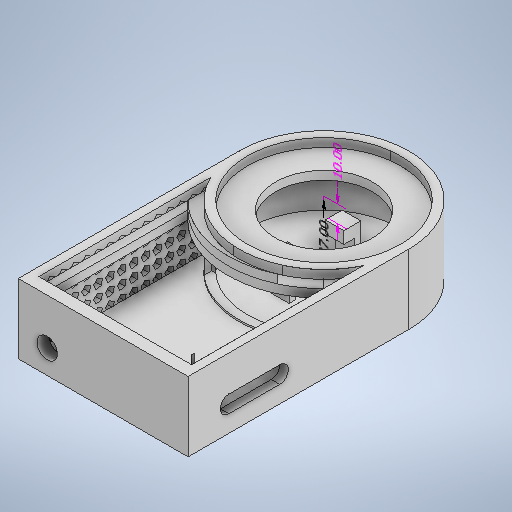
# Autodesk Inventor part: bazav2
Saved by Autodesk Inventor 2025.2 (Build 292293000, 293)
## iProperties
Created: 2025-08-28
Part Number: bazav2
Material: Ogólny
Document SubType Name: Modeling
Designer: IGOR
Density: 1 g/cm^3
Appearance: Domyślna
Author: IGOR
Autodesk Inventor part; units mm, degrees
ref_plane "YZ Plane" through (0, 0, 0) normal (1, 0, 0) x (0, 1, 0)
ref_plane "XZ Plane" through (0, 0, 0) normal (0, 1, 0) x (-1, 0, 0)
ref_plane "XY Plane" through (0, 0, 0) normal (0, 0, 1) x (1, 0, 0)
sketch "Szkic1" plane through (0, 0, 0) normal (0, 1, 0) x (-1, 0, 0)
  circle A0 centre (0.082273, -0.020568) radius 50
  circle A1 centre (0.082273, -0.020568) radius 45
  line L0 (-5.417727, 25.979432) -> (5.582273, 25.979432)
  line L1 (5.582273, 25.979432) -> (5.582273, 15.979432)
  line L2 (5.582273, 15.979432) -> (-5.417727, 15.979432)
  line L3 (-5.417727, 15.979432) -> (-5.417727, 25.979432)
  line L4 (-5.417727, 25.979432) -> (5.582273, 15.979432) construction
  line L5 (5.582273, 25.979432) -> (-5.417727, 15.979432) construction
  line L6 (-5.417727, -6.270568) -> (5.582273, -6.270568)
  line L7 (5.582273, -6.270568) -> (5.582273, -16.270568)
  line L8 (5.582273, -16.270568) -> (-5.417727, -16.270568)
  line L9 (-5.417727, -16.270568) -> (-5.417727, -6.270568)
  line L10 (-5.417727, -6.270568) -> (5.582273, -16.270568) construction
  line L11 (5.582273, -6.270568) -> (-5.417727, -16.270568) construction
  line L12 (50.082273, -0.020568) -> (50.082273, 129.979432)
  line L13 (50.082273, 129.979432) -> (-49.917727, 129.979432)
  line L14 (-49.917727, 129.979432) -> (-49.917727, -0.020568)
  line L15 (-17.866681, -46.687849) -> (50.082273, 129.979432) construction
  line L16 (18.031227, -46.687849) -> (-49.917727, 129.979432) construction
  line L17 (45.082273, -21.815063) -> (45.082273, 123)
  line L18 (45.082273, 123) -> (-44.917727, 123)
  line L19 (-44.917727, 123) -> (-44.917727, -21.815063)
  line L20 (-17.09427, -46.977638) -> (45.082273, 123) construction
  line L21 (17.258816, -46.977638) -> (-44.917727, 123) construction
  point P0 (0, 0)
  point P1 (0.082273, 20.979432)
  point P2 (0.082273, -11.270568)
  point P3 (0.082273, 15.979432)
  point P4 (45.082273, 21.773926)
  point P5 (-44.917727, 21.773926)
  dimension "d0" = 100
  dimension "d1" = 90
  dimension "d2" = 11
  dimension "d3" = 10
  dimension "d4" = 11
  dimension "d5" = 10
  dimension "d6" = 6.25
  dimension "d7" = 16
  constraints: 44 end point, 6 parallel, 5 midpoint, 4 point on line, 2 coincident, 2 horizontal, 2 perpendicular, 1 centre point, 10 other
  measures "d1" diameter of A1
  measures "d2" distance of L2.start L2.end
  measures "d3" distance of L5.start L2.start
  measures "d4" distance of L7.end L9.start
  measures "d5" distance of L6.end L7.end
  measures "d6" distance from line of point (0.082, -0.021) L6
  measures "d7" distance of point (0.082, 15.979) point (0.082, -0.021)
extrude "Wyciągnięcie proste1" add sketch "Szkic1" along normal blind 41 contours A0 L19 | L14 L13 L12 A0 L17 L18 L19 | L19 A1 L17 A0 | A0 L17 A1 L19 | L17 A0
extrude "Wyciągnięcie proste2" add sketch "Szkic1" along normal blind 4 contours L19 L18 L17 A0 | A1
extrude "Wyciągnięcie proste3" add sketch "Szkic1" along normal blind 25 contours L0 L1 L2 L3 | L6 L7 L8 L9
sketch "Szkic2" plane through (44.917727, 41, 123) normal (0, 0, -1) x (-1, 0, 0)
  line L0 (78, -36) -> (6, -36)
  line L1 (6, -36) -> (6, -10)
  line L2 (6, -10) -> (78, -10)
  line L3 (78, -10) -> (78, -36)
  point P0 (44.917727, -41)
  constraints: 8 end point, 2 parallel, 1 horizontal, 1 perpendicular
extrude "Wyciągnięcie proste4" cut sketch "Szkic2" along normal blind 90
sketch "Szkic3" plane through (0, 41, 0) normal (0, 1, 0) x (1, 0, 0)
  circle A0 centre (0, 0) radius 45.009943
  circle A1 centre (0, 0) radius 28.551038
  constraints: 2 centre point, 2 coincident
extrude "Wyciągnięcie proste5" add sketch "Szkic3" against normal blind 10
sketch "Szkic4" plane through (0, 41, 0) normal (0, 1, 0) x (1, 0, 0)
  circle A0 centre (0, 0) radius 45.03064
  circle A1 centre (0, 0) radius 28.551038
  constraints: 2 centre point, 2 coincident
extrude "Wyciągnięcie proste6" cut sketch "Szkic4" against normal blind 5
sketch "Szkic5" plane through (5.417727, 4, -16.270568) normal (1, 0, 0) x (0, 0, -1)
  line L0 (0, 0) -> (-10, 0) projected
  line L1 (-10, 0) -> (-4, 0)
  line L2 (-4, 0) -> (-4, 14)
  line L3 (-4, 14) -> (-10, 14)
  line L4 (-10, 14) -> (-10, 0)
  line L5 (-32.25, 0) -> (-42.25, 0) projected
  line L6 (-32.25, 0) -> (-38.25, 0)
  line L7 (-38.25, 0) -> (-38.25, 14)
  line L8 (-38.25, 14) -> (-32.25, 14)
  line L9 (-32.25, 14) -> (-32.25, 0)
  point P0 (-16.270568, -4)
  point P1 (-4, 0)
  point P2 (-38.25, 0)
  dimension "d23" = 6
  dimension "d24" = 14
  constraints: 16 end point, 4 parallel, 2 horizontal, 2 perpendicular
  measures "d23" distance of L7.end L8.end
  measures "d24" distance of L6.end L7.end
extrude "Wyciągnięcie proste7" cut sketch "Szkic5" against normal blind 11
sketch "Szkic6" plane through (0, 41, 0) normal (0, 1, 0) x (1, 0, 0)
  line L0 (44.917727, -21.773926) -> (44.917727, -123)
  line L1 (-45.082273, -123) -> (44.917727, -123)
  line L2 (44.917727, -123) -> (44.917727, -21.773926)
  line L3 (-45.025483, -21.773926) -> (-45.082273, -21.773926)
  line L4 (-45.082273, -21.773926) -> (-45.082273, -123)
  arc A0 (-45.025483, -21.773926) -> (44.917727, -21.995359) centre (0, 0) ccw
  arc A1 (-40.082273, -40.132904) -> (39.917727, -40.296572) centre (0, 0) ccw
  line L5 (-40.082273, -118) -> (39.917727, -118)
  line L6 (39.917727, -118) -> (39.917727, -40.296572)
  line L7 (-40.082273, -40.132904) -> (-40.082273, -118)
  point P0 (39.917727, -79.148286)
  point P1 (44.917727, -21.995359)
  dimension "d27" = 5
  dimension "d28" = 5
  dimension "d29" = 5
  dimension "d30" = 6.70673
  constraints: 14 end point, 4 point on circle, 3 parallel, 2 centre point, 2 coincident, 2 horizontal, 2 perpendicular, 1 midpoint, 1 point on line
  measures "d27" distance from line of point (39.918, -79.148) L0
  measures "d28" distance between parallel lines of L4 L7
  measures "d29" distance between parallel lines of L1 L5
  measures "d30" radial gap between concentric circles of A1 A0
extrude "Wyciągnięcie proste8" add sketch "Szkic6" against normal blind 10
sketch "Szkic7" plane through (0, 41, 0) normal (0, 1, 0) x (1, 0, 0)
  line L0 (44.972521, -21.748488) -> (44.972521, -122.974561)
  line L1 (-45.027479, -122.974561) -> (44.972521, -122.974561)
  line L2 (44.972521, -122.974561) -> (44.972521, -21.748488)
  line L3 (-44.970689, -21.748488) -> (-45.027479, -21.748488)
  line L4 (-45.027479, -21.748488) -> (-45.027479, -122.974561)
  arc A0 (-44.970689, -21.748488) -> (44.972521, -21.96992) centre (0.054794, 0.025439) ccw
  arc A1 (-40.027479, -40.107466) -> (39.972521, -40.271133) centre (0.054794, 0.025439) ccw
  line L5 (-40.027479, -117.974561) -> (39.972521, -117.974561)
  line L6 (39.972521, -117.974561) -> (39.972521, -40.271133)
  line L7 (-40.027479, -40.107466) -> (-40.027479, -117.974561)
  point P0 (0, 0)
  point P1 (39.972521, -79.122847)
  point P2 (44.972521, -21.96992)
  dimension "d33" = 5
  dimension "d34" = 5
  dimension "d35" = 5
  dimension "d36" = 6.70673
  constraints: 16 end point, 4 point on circle, 3 parallel, 2 centre point, 2 horizontal, 2 perpendicular, 1 coincident, 1 midpoint, 1 point on line
  measures "d33" distance from line of point (39.973, -79.123) L0
  measures "d34" distance between parallel lines of L4 L7
  measures "d35" distance between parallel lines of L1 L5
  measures "d36" radial gap between concentric circles of A1 A0
extrude "Wyciągnięcie proste9" cut sketch "Szkic7" against normal blind 5
sketch "Szkic8" plane through (39.917727, 31, 40.296572) normal (-1, 0, 0) x (0, 0, 1)
  line L0 (0.028766, 10) -> (77.677989, 10)
  line L1 (0, 5) -> (0, 0)
  line L2 (76, 10) -> (0, 10)
  line L3 (0, 10) -> (0, 5)
  line L4 (0, 5) -> (76, 5)
  line L5 (76, 5) -> (76, 10)
  point P0 (-40.296572, -31)
  constraints: 8 end point, 2 parallel, 1 horizontal, 1 perpendicular, 1 point on line
extrude "Wyciągnięcie proste10" cut sketch "Szkic8" against normal blind 1
sketch "Szkic9" plane through (-50.082273, 0, 129.979432) normal (0, 0, 1) x (1, 0, 0)
  line L0 (17, 5) -> (17, 31) projected
  circle A0 centre (17, 14) radius 6
  point P0 (50.082273, 0)
  dimension "d41" = 12
  constraints: 1 centre point, 1 point on line
  measures "d41" diameter of A0
extrude "Wyciągnięcie proste11" cut sketch "Szkic9" against normal blind 10
sketch "Szkic11" plane through (49.917727, 0, 129.979432) normal (1, 0, 0) x (0, 0, -1)
  line L0 (24, 15) -> (54, 15) construction
  line L1 (24, 10) -> (54, 10)
  line L2 (54, 20) -> (24, 20)
  arc A0 (24, 20) -> (24, 10) centre (24, 15) ccw
  arc A1 (54, 10) -> (54, 20) centre (54, 15) ccw
  point P0 (129.979432, 0)
  point P1 (39, 15)
  constraints: 8 end point, 4 point on circle, 4 tangent, 2 centre point, 1 horizontal, 1 midpoint, 1 parallel
extrude "Wyciągnięcie proste13" cut sketch "Szkic11" against normal blind 10
sketch "Szkic12" plane through (-50.082273, 0, -0.020568) normal (-1, 0, 0) x (0, 0, 1)
  line L0 (12.273457, 32.546915) -> (9.060497, 33.030825)
  line L1 (9.060497, 33.030825) -> (8.527864, 36.236068)
  line L2 (8.527864, 36.236068) -> (11.411638, 37.733107)
  line L3 (11.411638, 37.733107) -> (13.726543, 35.453085)
  line L4 (13.726543, 35.453085) -> (12.273457, 32.546915)
  line L5 (0, 0) -> (0, 41)
  line L6 (130, 0) -> (130, 41)
  line L7 (0, 41) -> (130, 41)
  line L8 (130, 41) -> (130, 0)
  line L9 (130, 0) -> (0, 0)
  line L10 (0, 0) -> (0, 41)
  line L11 (18.411638, 37.733107) -> (20.726543, 35.453085)
  line L12 (20.726543, 35.453085) -> (19.273457, 32.546915)
  line L13 (19.273457, 32.546915) -> (16.060497, 33.030825)
  line L14 (16.060497, 33.030825) -> (15.527864, 36.236068)
  line L15 (15.527864, 36.236068) -> (18.411638, 37.733107)
  line L16 (25.411638, 37.733107) -> (27.726543, 35.453085)
  line L17 (27.726543, 35.453085) -> (26.273457, 32.546915)
  line L18 (26.273457, 32.546915) -> (23.060497, 33.030825)
  line L19 (23.060497, 33.030825) -> (22.527864, 36.236068)
  line L20 (22.527864, 36.236068) -> (25.411638, 37.733107)
  line L21 (32.411638, 37.733107) -> (34.726543, 35.453085)
  line L22 (34.726543, 35.453085) -> (33.273457, 32.546915)
  line L23 (33.273457, 32.546915) -> (30.060497, 33.030825)
  line L24 (30.060497, 33.030825) -> (29.527864, 36.236068)
  line L25 (29.527864, 36.236068) -> (32.411638, 37.733107)
  line L26 (39.411638, 37.733107) -> (41.726543, 35.453085)
  line L27 (41.726543, 35.453085) -> (40.273457, 32.546915)
  line L28 (40.273457, 32.546915) -> (37.060497, 33.030825)
  line L29 (37.060497, 33.030825) -> (36.527864, 36.236068)
  line L30 (36.527864, 36.236068) -> (39.411638, 37.733107)
  line L31 (46.411638, 37.733107) -> (48.726543, 35.453085)
  line L32 (48.726543, 35.453085) -> (47.273457, 32.546915)
  line L33 (47.273457, 32.546915) -> (44.060497, 33.030825)
  line L34 (44.060497, 33.030825) -> (43.527864, 36.236068)
  line L35 (43.527864, 36.236068) -> (46.411638, 37.733107)
  line L36 (53.411638, 37.733107) -> (55.726543, 35.453085)
  line L37 (55.726543, 35.453085) -> (54.273457, 32.546915)
  line L38 (54.273457, 32.546915) -> (51.060497, 33.030825)
  line L39 (51.060497, 33.030825) -> (50.527864, 36.236068)
  line L40 (50.527864, 36.236068) -> (53.411638, 37.733107)
  line L41 (60.411638, 37.733107) -> (62.726543, 35.453085)
  line L42 (62.726543, 35.453085) -> (61.273457, 32.546915)
  line L43 (61.273457, 32.546915) -> (58.060497, 33.030825)
  line L44 (58.060497, 33.030825) -> (57.527864, 36.236068)
  line L45 (57.527864, 36.236068) -> (60.411638, 37.733107)
  line L46 (67.411638, 37.733107) -> (69.726543, 35.453085)
  line L47 (69.726543, 35.453085) -> (68.273457, 32.546915)
  line L48 (68.273457, 32.546915) -> (65.060497, 33.030825)
  line L49 (65.060497, 33.030825) -> (64.527864, 36.236068)
  line L50 (64.527864, 36.236068) -> (67.411638, 37.733107)
  line L51 (74.411638, 37.733107) -> (76.726543, 35.453085)
  line L52 (76.726543, 35.453085) -> (75.273457, 32.546915)
  line L53 (75.273457, 32.546915) -> (72.060497, 33.030825)
  line L54 (72.060497, 33.030825) -> (71.527864, 36.236068)
  line L55 (71.527864, 36.236068) -> (74.411638, 37.733107)
  line L56 (81.411638, 37.733107) -> (83.726543, 35.453085)
  line L57 (83.726543, 35.453085) -> (82.273457, 32.546915)
  line L58 (82.273457, 32.546915) -> (79.060497, 33.030825)
  line L59 (79.060497, 33.030825) -> (78.527864, 36.236068)
  line L60 (78.527864, 36.236068) -> (81.411638, 37.733107)
  line L61 (88.411638, 37.733107) -> (90.726543, 35.453085)
  line L62 (90.726543, 35.453085) -> (89.273457, 32.546915)
  line L63 (89.273457, 32.546915) -> (86.060497, 33.030825)
  line L64 (86.060497, 33.030825) -> (85.527864, 36.236068)
  line L65 (85.527864, 36.236068) -> (88.411638, 37.733107)
  line L66 (95.411638, 37.733107) -> (97.726543, 35.453085)
  line L67 (97.726543, 35.453085) -> (96.273457, 32.546915)
  line L68 (96.273457, 32.546915) -> (93.060497, 33.030825)
  line L69 (93.060497, 33.030825) -> (92.527864, 36.236068)
  line L70 (92.527864, 36.236068) -> (95.411638, 37.733107)
  line L71 (102.411638, 37.733107) -> (104.726543, 35.453085)
  line L72 (104.726543, 35.453085) -> (103.273457, 32.546915)
  line L73 (103.273457, 32.546915) -> (100.060497, 33.030825)
  line L74 (100.060497, 33.030825) -> (99.527864, 36.236068)
  line L75 (99.527864, 36.236068) -> (102.411638, 37.733107)
  line L76 (109.411638, 37.733107) -> (111.726543, 35.453085)
  line L77 (111.726543, 35.453085) -> (110.273457, 32.546915)
  line L78 (110.273457, 32.546915) -> (107.060497, 33.030825)
  line L79 (107.060497, 33.030825) -> (106.527864, 36.236068)
  line L80 (106.527864, 36.236068) -> (109.411638, 37.733107)
  line L81 (116.411638, 37.733107) -> (118.726543, 35.453085)
  line L82 (118.726543, 35.453085) -> (117.273457, 32.546915)
  line L83 (117.273457, 32.546915) -> (114.060497, 33.030825)
  line L84 (114.060497, 33.030825) -> (113.527864, 36.236068)
  line L85 (113.527864, 36.236068) -> (116.411638, 37.733107)
  line L86 (123.411638, 37.733107) -> (125.726543, 35.453085)
  line L87 (125.726543, 35.453085) -> (124.273457, 32.546915)
  line L88 (124.273457, 32.546915) -> (121.060497, 33.030825)
  line L89 (121.060497, 33.030825) -> (120.527864, 36.236068)
  line L90 (120.527864, 36.236068) -> (123.411638, 37.733107)
  line L91 (11.411638, 30.233107) -> (13.726543, 27.953085)
  line L92 (13.726543, 27.953085) -> (12.273457, 25.046915)
  line L93 (12.273457, 25.046915) -> (9.060497, 25.530825)
  line L94 (9.060497, 25.530825) -> (8.527864, 28.736068)
  line L95 (8.527864, 28.736068) -> (11.411638, 30.233107)
  line L96 (18.411638, 30.233107) -> (20.726543, 27.953085)
  line L97 (20.726543, 27.953085) -> (19.273457, 25.046915)
  line L98 (19.273457, 25.046915) -> (16.060497, 25.530825)
  line L99 (16.060497, 25.530825) -> (15.527864, 28.736068)
  line L100 (15.527864, 28.736068) -> (18.411638, 30.233107)
  line L101 (25.411638, 30.233107) -> (27.726543, 27.953085)
  line L102 (27.726543, 27.953085) -> (26.273457, 25.046915)
  line L103 (26.273457, 25.046915) -> (23.060497, 25.530825)
  line L104 (23.060497, 25.530825) -> (22.527864, 28.736068)
  line L105 (22.527864, 28.736068) -> (25.411638, 30.233107)
  line L106 (32.411638, 30.233107) -> (34.726543, 27.953085)
  line L107 (34.726543, 27.953085) -> (33.273457, 25.046915)
  line L108 (33.273457, 25.046915) -> (30.060497, 25.530825)
  line L109 (30.060497, 25.530825) -> (29.527864, 28.736068)
  line L110 (29.527864, 28.736068) -> (32.411638, 30.233107)
  line L111 (39.411638, 30.233107) -> (41.726543, 27.953085)
  line L112 (41.726543, 27.953085) -> (40.273457, 25.046915)
  line L113 (40.273457, 25.046915) -> (37.060497, 25.530825)
  line L114 (37.060497, 25.530825) -> (36.527864, 28.736068)
  line L115 (36.527864, 28.736068) -> (39.411638, 30.233107)
  line L116 (46.411638, 30.233107) -> (48.726543, 27.953085)
  line L117 (48.726543, 27.953085) -> (47.273457, 25.046915)
  line L118 (47.273457, 25.046915) -> (44.060497, 25.530825)
  line L119 (44.060497, 25.530825) -> (43.527864, 28.736068)
  line L120 (43.527864, 28.736068) -> (46.411638, 30.233107)
  line L121 (53.411638, 30.233107) -> (55.726543, 27.953085)
  line L122 (55.726543, 27.953085) -> (54.273457, 25.046915)
  line L123 (54.273457, 25.046915) -> (51.060497, 25.530825)
  line L124 (51.060497, 25.530825) -> (50.527864, 28.736068)
  line L125 (50.527864, 28.736068) -> (53.411638, 30.233107)
  line L126 (60.411638, 30.233107) -> (62.726543, 27.953085)
  line L127 (62.726543, 27.953085) -> (61.273457, 25.046915)
  line L128 (61.273457, 25.046915) -> (58.060497, 25.530825)
  line L129 (58.060497, 25.530825) -> (57.527864, 28.736068)
  line L130 (57.527864, 28.736068) -> (60.411638, 30.233107)
  line L131 (67.411638, 30.233107) -> (69.726543, 27.953085)
  line L132 (69.726543, 27.953085) -> (68.273457, 25.046915)
  line L133 (68.273457, 25.046915) -> (65.060497, 25.530825)
  line L134 (65.060497, 25.530825) -> (64.527864, 28.736068)
  line L135 (64.527864, 28.736068) -> (67.411638, 30.233107)
  line L136 (74.411638, 30.233107) -> (76.726543, 27.953085)
  line L137 (76.726543, 27.953085) -> (75.273457, 25.046915)
  line L138 (75.273457, 25.046915) -> (72.060497, 25.530825)
  line L139 (72.060497, 25.530825) -> (71.527864, 28.736068)
  line L140 (71.527864, 28.736068) -> (74.411638, 30.233107)
  line L141 (81.411638, 30.233107) -> (83.726543, 27.953085)
  line L142 (83.726543, 27.953085) -> (82.273457, 25.046915)
  line L143 (82.273457, 25.046915) -> (79.060497, 25.530825)
  line L144 (79.060497, 25.530825) -> (78.527864, 28.736068)
  line L145 (78.527864, 28.736068) -> (81.411638, 30.233107)
  line L146 (88.411638, 30.233107) -> (90.726543, 27.953085)
  line L147 (90.726543, 27.953085) -> (89.273457, 25.046915)
  line L148 (89.273457, 25.046915) -> (86.060497, 25.530825)
  line L149 (86.060497, 25.530825) -> (85.527864, 28.736068)
  line L150 (85.527864, 28.736068) -> (88.411638, 30.233107)
  line L151 (95.411638, 30.233107) -> (97.726543, 27.953085)
  line L152 (97.726543, 27.953085) -> (96.273457, 25.046915)
  line L153 (96.273457, 25.046915) -> (93.060497, 25.530825)
  line L154 (93.060497, 25.530825) -> (92.527864, 28.736068)
  line L155 (92.527864, 28.736068) -> (95.411638, 30.233107)
  line L156 (102.411638, 30.233107) -> (104.726543, 27.953085)
  line L157 (104.726543, 27.953085) -> (103.273457, 25.046915)
  line L158 (103.273457, 25.046915) -> (100.060497, 25.530825)
  line L159 (100.060497, 25.530825) -> (99.527864, 28.736068)
  line L160 (99.527864, 28.736068) -> (102.411638, 30.233107)
  line L161 (109.411638, 30.233107) -> (111.726543, 27.953085)
  line L162 (111.726543, 27.953085) -> (110.273457, 25.046915)
  line L163 (110.273457, 25.046915) -> (107.060497, 25.530825)
  line L164 (107.060497, 25.530825) -> (106.527864, 28.736068)
  line L165 (106.527864, 28.736068) -> (109.411638, 30.233107)
  line L166 (116.411638, 30.233107) -> (118.726543, 27.953085)
  line L167 (118.726543, 27.953085) -> (117.273457, 25.046915)
  line L168 (117.273457, 25.046915) -> (114.060497, 25.530825)
  line L169 (114.060497, 25.530825) -> (113.527864, 28.736068)
  line L170 (113.527864, 28.736068) -> (116.411638, 30.233107)
  line L171 (123.411638, 30.233107) -> (125.726543, 27.953085)
  line L172 (125.726543, 27.953085) -> (124.273457, 25.046915)
  line L173 (124.273457, 25.046915) -> (121.060497, 25.530825)
  line L174 (121.060497, 25.530825) -> (120.527864, 28.736068)
  line L175 (120.527864, 28.736068) -> (123.411638, 30.233107)
  line L176 (11.411638, 22.733107) -> (13.726543, 20.453085)
  line L177 (13.726543, 20.453085) -> (12.273457, 17.546915)
  line L178 (12.273457, 17.546915) -> (9.060497, 18.030825)
  line L179 (9.060497, 18.030825) -> (8.527864, 21.236068)
  line L180 (8.527864, 21.236068) -> (11.411638, 22.733107)
  line L181 (18.411638, 22.733107) -> (20.726543, 20.453085)
  line L182 (20.726543, 20.453085) -> (19.273457, 17.546915)
  line L183 (19.273457, 17.546915) -> (16.060497, 18.030825)
  line L184 (16.060497, 18.030825) -> (15.527864, 21.236068)
  line L185 (15.527864, 21.236068) -> (18.411638, 22.733107)
  line L186 (25.411638, 22.733107) -> (27.726543, 20.453085)
  line L187 (27.726543, 20.453085) -> (26.273457, 17.546915)
  line L188 (26.273457, 17.546915) -> (23.060497, 18.030825)
  line L189 (23.060497, 18.030825) -> (22.527864, 21.236068)
  line L190 (22.527864, 21.236068) -> (25.411638, 22.733107)
  line L191 (32.411638, 22.733107) -> (34.726543, 20.453085)
  line L192 (34.726543, 20.453085) -> (33.273457, 17.546915)
  line L193 (33.273457, 17.546915) -> (30.060497, 18.030825)
  line L194 (30.060497, 18.030825) -> (29.527864, 21.236068)
  line L195 (29.527864, 21.236068) -> (32.411638, 22.733107)
  line L196 (39.411638, 22.733107) -> (41.726543, 20.453085)
  line L197 (41.726543, 20.453085) -> (40.273457, 17.546915)
  line L198 (40.273457, 17.546915) -> (37.060497, 18.030825)
  line L199 (37.060497, 18.030825) -> (36.527864, 21.236068)
  line L200 (36.527864, 21.236068) -> (39.411638, 22.733107)
  line L201 (46.411638, 22.733107) -> (48.726543, 20.453085)
  line L202 (48.726543, 20.453085) -> (47.273457, 17.546915)
  line L203 (47.273457, 17.546915) -> (44.060497, 18.030825)
  line L204 (44.060497, 18.030825) -> (43.527864, 21.236068)
  line L205 (43.527864, 21.236068) -> (46.411638, 22.733107)
  line L206 (53.411638, 22.733107) -> (55.726543, 20.453085)
  line L207 (55.726543, 20.453085) -> (54.273457, 17.546915)
  line L208 (54.273457, 17.546915) -> (51.060497, 18.030825)
  line L209 (51.060497, 18.030825) -> (50.527864, 21.236068)
  line L210 (50.527864, 21.236068) -> (53.411638, 22.733107)
  line L211 (60.411638, 22.733107) -> (62.726543, 20.453085)
  line L212 (62.726543, 20.453085) -> (61.273457, 17.546915)
  line L213 (61.273457, 17.546915) -> (58.060497, 18.030825)
  line L214 (58.060497, 18.030825) -> (57.527864, 21.236068)
  line L215 (57.527864, 21.236068) -> (60.411638, 22.733107)
  line L216 (67.411638, 22.733107) -> (69.726543, 20.453085)
  line L217 (69.726543, 20.453085) -> (68.273457, 17.546915)
  line L218 (68.273457, 17.546915) -> (65.060497, 18.030825)
  line L219 (65.060497, 18.030825) -> (64.527864, 21.236068)
  line L220 (64.527864, 21.236068) -> (67.411638, 22.733107)
  line L221 (74.411638, 22.733107) -> (76.726543, 20.453085)
  line L222 (76.726543, 20.453085) -> (75.273457, 17.546915)
  line L223 (75.273457, 17.546915) -> (72.060497, 18.030825)
  line L224 (72.060497, 18.030825) -> (71.527864, 21.236068)
  line L225 (71.527864, 21.236068) -> (74.411638, 22.733107)
  line L226 (81.411638, 22.733107) -> (83.726543, 20.453085)
  line L227 (83.726543, 20.453085) -> (82.273457, 17.546915)
  line L228 (82.273457, 17.546915) -> (79.060497, 18.030825)
  line L229 (79.060497, 18.030825) -> (78.527864, 21.236068)
  line L230 (78.527864, 21.236068) -> (81.411638, 22.733107)
  line L231 (88.411638, 22.733107) -> (90.726543, 20.453085)
  line L232 (90.726543, 20.453085) -> (89.273457, 17.546915)
  line L233 (89.273457, 17.546915) -> (86.060497, 18.030825)
  line L234 (86.060497, 18.030825) -> (85.527864, 21.236068)
  line L235 (85.527864, 21.236068) -> (88.411638, 22.733107)
  line L236 (95.411638, 22.733107) -> (97.726543, 20.453085)
  line L237 (97.726543, 20.453085) -> (96.273457, 17.546915)
  line L238 (96.273457, 17.546915) -> (93.060497, 18.030825)
  line L239 (93.060497, 18.030825) -> (92.527864, 21.236068)
  line L240 (92.527864, 21.236068) -> (95.411638, 22.733107)
  line L241 (102.411638, 22.733107) -> (104.726543, 20.453085)
  line L242 (104.726543, 20.453085) -> (103.273457, 17.546915)
  line L243 (103.273457, 17.546915) -> (100.060497, 18.030825)
  line L244 (100.060497, 18.030825) -> (99.527864, 21.236068)
  line L245 (99.527864, 21.236068) -> (102.411638, 22.733107)
  line L246 (109.411638, 22.733107) -> (111.726543, 20.453085)
  line L247 (111.726543, 20.453085) -> (110.273457, 17.546915)
  line L248 (110.273457, 17.546915) -> (107.060497, 18.030825)
  line L249 (107.060497, 18.030825) -> (106.527864, 21.236068)
  line L250 (106.527864, 21.236068) -> (109.411638, 22.733107)
  line L251 (116.411638, 22.733107) -> (118.726543, 20.453085)
  line L252 (118.726543, 20.453085) -> (117.273457, 17.546915)
  line L253 (117.273457, 17.546915) -> (114.060497, 18.030825)
  line L254 (114.060497, 18.030825) -> (113.527864, 21.236068)
  line L255 (113.527864, 21.236068) -> (116.411638, 22.733107)
  line L256 (123.411638, 22.733107) -> (125.726543, 20.453085)
  line L257 (125.726543, 20.453085) -> (124.273457, 17.546915)
  line L258 (124.273457, 17.546915) -> (121.060497, 18.030825)
  line L259 (121.060497, 18.030825) -> (120.527864, 21.236068)
  line L260 (120.527864, 21.236068) -> (123.411638, 22.733107)
  line L261 (11.411638, 15.233107) -> (13.726543, 12.953085)
  line L262 (13.726543, 12.953085) -> (12.273457, 10.046915)
  line L263 (12.273457, 10.046915) -> (9.060497, 10.530825)
  line L264 (9.060497, 10.530825) -> (8.527864, 13.736068)
  line L265 (8.527864, 13.736068) -> (11.411638, 15.233107)
  line L266 (18.411638, 15.233107) -> (20.726543, 12.953085)
  line L267 (20.726543, 12.953085) -> (19.273457, 10.046915)
  line L268 (19.273457, 10.046915) -> (16.060497, 10.530825)
  line L269 (16.060497, 10.530825) -> (15.527864, 13.736068)
  line L270 (15.527864, 13.736068) -> (18.411638, 15.233107)
  line L271 (25.411638, 15.233107) -> (27.726543, 12.953085)
  line L272 (27.726543, 12.953085) -> (26.273457, 10.046915)
  line L273 (26.273457, 10.046915) -> (23.060497, 10.530825)
  line L274 (23.060497, 10.530825) -> (22.527864, 13.736068)
  line L275 (22.527864, 13.736068) -> (25.411638, 15.233107)
  line L276 (32.411638, 15.233107) -> (34.726543, 12.953085)
  line L277 (34.726543, 12.953085) -> (33.273457, 10.046915)
  line L278 (33.273457, 10.046915) -> (30.060497, 10.530825)
  line L279 (30.060497, 10.530825) -> (29.527864, 13.736068)
  line L280 (29.527864, 13.736068) -> (32.411638, 15.233107)
  line L281 (39.411638, 15.233107) -> (41.726543, 12.953085)
  line L282 (41.726543, 12.953085) -> (40.273457, 10.046915)
  line L283 (40.273457, 10.046915) -> (37.060497, 10.530825)
  line L284 (37.060497, 10.530825) -> (36.527864, 13.736068)
  line L285 (36.527864, 13.736068) -> (39.411638, 15.233107)
  line L286 (46.411638, 15.233107) -> (48.726543, 12.953085)
  line L287 (48.726543, 12.953085) -> (47.273457, 10.046915)
  line L288 (47.273457, 10.046915) -> (44.060497, 10.530825)
  line L289 (44.060497, 10.530825) -> (43.527864, 13.736068)
  line L290 (43.527864, 13.736068) -> (46.411638, 15.233107)
  line L291 (53.411638, 15.233107) -> (55.726543, 12.953085)
  line L292 (55.726543, 12.953085) -> (54.273457, 10.046915)
  line L293 (54.273457, 10.046915) -> (51.060497, 10.530825)
  line L294 (51.060497, 10.530825) -> (50.527864, 13.736068)
  line L295 (50.527864, 13.736068) -> (53.411638, 15.233107)
  line L296 (60.411638, 15.233107) -> (62.726543, 12.953085)
  line L297 (62.726543, 12.953085) -> (61.273457, 10.046915)
  line L298 (61.273457, 10.046915) -> (58.060497, 10.530825)
  line L299 (58.060497, 10.530825) -> (57.527864, 13.736068)
  line L300 (57.527864, 13.736068) -> (60.411638, 15.233107)
  line L301 (67.411638, 15.233107) -> (69.726543, 12.953085)
  line L302 (69.726543, 12.953085) -> (68.273457, 10.046915)
  line L303 (68.273457, 10.046915) -> (65.060497, 10.530825)
  line L304 (65.060497, 10.530825) -> (64.527864, 13.736068)
  line L305 (64.527864, 13.736068) -> (67.411638, 15.233107)
  line L306 (74.411638, 15.233107) -> (76.726543, 12.953085)
  line L307 (76.726543, 12.953085) -> (75.273457, 10.046915)
  line L308 (75.273457, 10.046915) -> (72.060497, 10.530825)
  line L309 (72.060497, 10.530825) -> (71.527864, 13.736068)
  line L310 (71.527864, 13.736068) -> (74.411638, 15.233107)
  line L311 (81.411638, 15.233107) -> (83.726543, 12.953085)
  line L312 (83.726543, 12.953085) -> (82.273457, 10.046915)
  line L313 (82.273457, 10.046915) -> (79.060497, 10.530825)
  line L314 (79.060497, 10.530825) -> (78.527864, 13.736068)
  line L315 (78.527864, 13.736068) -> (81.411638, 15.233107)
  line L316 (88.411638, 15.233107) -> (90.726543, 12.953085)
  line L317 (90.726543, 12.953085) -> (89.273457, 10.046915)
  line L318 (89.273457, 10.046915) -> (86.060497, 10.530825)
  line L319 (86.060497, 10.530825) -> (85.527864, 13.736068)
  line L320 (85.527864, 13.736068) -> (88.411638, 15.233107)
  line L321 (95.411638, 15.233107) -> (97.726543, 12.953085)
  line L322 (97.726543, 12.953085) -> (96.273457, 10.046915)
  line L323 (96.273457, 10.046915) -> (93.060497, 10.530825)
  line L324 (93.060497, 10.530825) -> (92.527864, 13.736068)
  line L325 (92.527864, 13.736068) -> (95.411638, 15.233107)
  line L326 (102.411638, 15.233107) -> (104.726543, 12.953085)
  line L327 (104.726543, 12.953085) -> (103.273457, 10.046915)
  line L328 (103.273457, 10.046915) -> (100.060497, 10.530825)
  line L329 (100.060497, 10.530825) -> (99.527864, 13.736068)
  line L330 (99.527864, 13.736068) -> (102.411638, 15.233107)
  line L331 (109.411638, 15.233107) -> (111.726543, 12.953085)
  line L332 (111.726543, 12.953085) -> (110.273457, 10.046915)
  line L333 (110.273457, 10.046915) -> (107.060497, 10.530825)
  line L334 (107.060497, 10.530825) -> (106.527864, 13.736068)
  line L335 (106.527864, 13.736068) -> (109.411638, 15.233107)
  line L336 (116.411638, 15.233107) -> (118.726543, 12.953085)
  line L337 (118.726543, 12.953085) -> (117.273457, 10.046915)
  line L338 (117.273457, 10.046915) -> (114.060497, 10.530825)
  line L339 (114.060497, 10.530825) -> (113.527864, 13.736068)
  line L340 (113.527864, 13.736068) -> (116.411638, 15.233107)
  line L341 (123.411638, 15.233107) -> (125.726543, 12.953085)
  line L342 (125.726543, 12.953085) -> (124.273457, 10.046915)
  line L343 (124.273457, 10.046915) -> (121.060497, 10.530825)
  line L344 (121.060497, 10.530825) -> (120.527864, 13.736068)
  line L345 (120.527864, 13.736068) -> (123.411638, 15.233107)
  line L346 (11.411638, 7.733107) -> (13.726543, 5.453085)
  line L347 (13.726543, 5.453085) -> (12.273457, 2.546915)
  line L348 (12.273457, 2.546915) -> (9.060497, 3.030825)
  line L349 (9.060497, 3.030825) -> (8.527864, 6.236068)
  line L350 (8.527864, 6.236068) -> (11.411638, 7.733107)
  line L351 (18.411638, 7.733107) -> (20.726543, 5.453085)
  line L352 (20.726543, 5.453085) -> (19.273457, 2.546915)
  line L353 (19.273457, 2.546915) -> (16.060497, 3.030825)
  line L354 (16.060497, 3.030825) -> (15.527864, 6.236068)
  line L355 (15.527864, 6.236068) -> (18.411638, 7.733107)
  line L356 (25.411638, 7.733107) -> (27.726543, 5.453085)
  line L357 (27.726543, 5.453085) -> (26.273457, 2.546915)
  line L358 (26.273457, 2.546915) -> (23.060497, 3.030825)
  line L359 (23.060497, 3.030825) -> (22.527864, 6.236068)
  line L360 (22.527864, 6.236068) -> (25.411638, 7.733107)
  line L361 (32.411638, 7.733107) -> (34.726543, 5.453085)
  line L362 (34.726543, 5.453085) -> (33.273457, 2.546915)
  line L363 (33.273457, 2.546915) -> (30.060497, 3.030825)
  line L364 (30.060497, 3.030825) -> (29.527864, 6.236068)
  line L365 (29.527864, 6.236068) -> (32.411638, 7.733107)
  line L366 (39.411638, 7.733107) -> (41.726543, 5.453085)
  line L367 (41.726543, 5.453085) -> (40.273457, 2.546915)
  line L368 (40.273457, 2.546915) -> (37.060497, 3.030825)
  line L369 (37.060497, 3.030825) -> (36.527864, 6.236068)
  line L370 (36.527864, 6.236068) -> (39.411638, 7.733107)
  line L371 (46.411638, 7.733107) -> (48.726543, 5.453085)
  line L372 (48.726543, 5.453085) -> (47.273457, 2.546915)
  line L373 (47.273457, 2.546915) -> (44.060497, 3.030825)
  line L374 (44.060497, 3.030825) -> (43.527864, 6.236068)
  line L375 (43.527864, 6.236068) -> (46.411638, 7.733107)
  line L376 (53.411638, 7.733107) -> (55.726543, 5.453085)
  line L377 (55.726543, 5.453085) -> (54.273457, 2.546915)
  line L378 (54.273457, 2.546915) -> (51.060497, 3.030825)
  line L379 (51.060497, 3.030825) -> (50.527864, 6.236068)
  line L380 (50.527864, 6.236068) -> (53.411638, 7.733107)
  line L381 (60.411638, 7.733107) -> (62.726543, 5.453085)
  line L382 (62.726543, 5.453085) -> (61.273457, 2.546915)
  line L383 (61.273457, 2.546915) -> (58.060497, 3.030825)
  line L384 (58.060497, 3.030825) -> (57.527864, 6.236068)
  line L385 (57.527864, 6.236068) -> (60.411638, 7.733107)
  line L386 (67.411638, 7.733107) -> (69.726543, 5.453085)
  line L387 (69.726543, 5.453085) -> (68.273457, 2.546915)
  line L388 (68.273457, 2.546915) -> (65.060497, 3.030825)
  line L389 (65.060497, 3.030825) -> (64.527864, 6.236068)
  line L390 (64.527864, 6.236068) -> (67.411638, 7.733107)
  line L391 (74.411638, 7.733107) -> (76.726543, 5.453085)
  line L392 (76.726543, 5.453085) -> (75.273457, 2.546915)
  line L393 (75.273457, 2.546915) -> (72.060497, 3.030825)
  line L394 (72.060497, 3.030825) -> (71.527864, 6.236068)
  line L395 (71.527864, 6.236068) -> (74.411638, 7.733107)
  line L396 (81.411638, 7.733107) -> (83.726543, 5.453085)
  line L397 (83.726543, 5.453085) -> (82.273457, 2.546915)
  line L398 (82.273457, 2.546915) -> (79.060497, 3.030825)
  line L399 (79.060497, 3.030825) -> (78.527864, 6.236068)
  line L400 (78.527864, 6.236068) -> (81.411638, 7.733107)
  line L401 (88.411638, 7.733107) -> (90.726543, 5.453085)
  line L402 (90.726543, 5.453085) -> (89.273457, 2.546915)
  line L403 (89.273457, 2.546915) -> (86.060497, 3.030825)
  line L404 (86.060497, 3.030825) -> (85.527864, 6.236068)
  line L405 (85.527864, 6.236068) -> (88.411638, 7.733107)
  line L406 (95.411638, 7.733107) -> (97.726543, 5.453085)
  line L407 (97.726543, 5.453085) -> (96.273457, 2.546915)
  line L408 (96.273457, 2.546915) -> (93.060497, 3.030825)
  line L409 (93.060497, 3.030825) -> (92.527864, 6.236068)
  line L410 (92.527864, 6.236068) -> (95.411638, 7.733107)
  line L411 (102.411638, 7.733107) -> (104.726543, 5.453085)
  line L412 (104.726543, 5.453085) -> (103.273457, 2.546915)
  line L413 (103.273457, 2.546915) -> (100.060497, 3.030825)
  line L414 (100.060497, 3.030825) -> (99.527864, 6.236068)
  line L415 (99.527864, 6.236068) -> (102.411638, 7.733107)
  line L416 (109.411638, 7.733107) -> (111.726543, 5.453085)
  line L417 (111.726543, 5.453085) -> (110.273457, 2.546915)
  line L418 (110.273457, 2.546915) -> (107.060497, 3.030825)
  line L419 (107.060497, 3.030825) -> (106.527864, 6.236068)
  line L420 (106.527864, 6.236068) -> (109.411638, 7.733107)
  line L421 (116.411638, 7.733107) -> (118.726543, 5.453085)
  line L422 (118.726543, 5.453085) -> (117.273457, 2.546915)
  line L423 (117.273457, 2.546915) -> (114.060497, 3.030825)
  line L424 (114.060497, 3.030825) -> (113.527864, 6.236068)
  line L425 (113.527864, 6.236068) -> (116.411638, 7.733107)
  line L426 (123.411638, 7.733107) -> (125.726543, 5.453085)
  line L427 (125.726543, 5.453085) -> (124.273457, 2.546915)
  line L428 (124.273457, 2.546915) -> (121.060497, 3.030825)
  line L429 (121.060497, 3.030825) -> (120.527864, 6.236068)
  line L430 (120.527864, 6.236068) -> (123.411638, 7.733107)
  point P0 (0.020568, 0)
  point P1 (11, 35)
  dimension "d50" = 7
  dimension "d53" = 7.5
  constraints: 858 end point, 2 horizontal, 2 parallel, 1 perpendicular, 1 vertical, 851 other
  measures "d50" distance of L2.end L11.start
  measures "d53" distance of L2.end L91.start
extrude "Wyciągnięcie proste14" cut sketch "Szkic12" against normal blind 5 contours L0 L1 L2 L3 L4 | L11 L12 L13 L14 L15 | L16 L17 L18 L19 L20 | L21 L22 L23 L24 L25 | L26 L27 L28 L29 L30 | L31 L32 L33 L34 L35 | L36 L37 L38 L39 L40 | L41 L42 L43 L44 L45 | L46 L47 L48 L49 L50 | L51 L52 L53 L54 L55 | L56 L57 L58 L59 L60 | L61 L62 L63 L64 L65 | L66 L67 L68 L69 L70 | L71 L72 L73 L74 L75 | L76 L77 L78 L79 L80 | L81 L82 L83 L84 L85 | L86 L87 L88 L89 L90 | L91 L92 L93 L94 L95 | L96 L97 L98 L99 L100 | L101 L102 L103 L104 L105 | L106 L107 L108 L109 L110 | L111 L112 L113 L114 L115 | L116 L117 L118 L119 L120 | L121 L122 L123 L124 L125 | L126 L127 L128 L129 L130 | L131 L132 L133 L134 L135 | L136 L137 L138 L139 L140 | L141 L142 L143 L144 L145 | L146 L147 L148 L149 L150 | L151 L152 L153 L154 L155 | L156 L157 L158 L159 L160 | L161 L162 L163 L164 L165 | L166 L167 L168 L169 L170 | L171 L172 L173 L174 L175 | L176 L177 L178 L179 L180 | L181 L182 L183 L184 L185 | L186 L187 L188 L189 L190 | L191 L192 L193 L194 L195 | L196 L197 L198 L199 L200 | L201 L202 L203 L204 L205 | L206 L207 L208 L209 L210 | L211 L212 L213 L214 L215 | L216 L217 L218 L219 L220 | L221 L222 L223 L224 L225 | L226 L227 L228 L229 L230 | L231 L232 L233 L234 L235 | L236 L237 L238 L239 L240 | L241 L242 L243 L244 L245 | L246 L247 L248 L249 L250 | L251 L252 L253 L254 L255 | L256 L257 L258 L259 L260 | L261 L262 L263 L264 L265 | L266 L267 L268 L269 L270 | L271 L272 L273 L274 L275 | L276 L277 L278 L279 L280 | L281 L282 L283 L284 L285 | L286 L287 L288 L289 L290 | L291 L292 L293 L294 L295 | L296 L297 L298 L299 L300 | L301 L302 L303 L304 L305 | L306 L307 L308 L309 L310 | L311 L312 L313 L314 L315 | L316 L317 L318 L319 L320 | L321 L322 L323 L324 L325 | L326 L327 L328 L329 L330 | L331 L332 L333 L334 L335 | L336 L337 L338 L339 L340 | L341 L342 L343 L344 L345 | L346 L347 L348 L349 L350 | L351 L352 L353 L354 L355 | L356 L357 L358 L359 L360 | L361 L362 L363 L364 L365 | L366 L367 L368 L369 L370 | L371 L372 L373 L374 L375 | L376 L377 L378 L379 L380 | L381 L382 L383 L384 L385 | L386 L387 L388 L389 L390 | L391 L392 L393 L394 L395 | L396 L397 L398 L399 L400 | L401 L402 L403 L404 L405 | L406 L407 L408 L409 L410 | L411 L412 L413 L414 L415 | L416 L417 L418 L419 L420 | L421 L422 L423 L424 L425 | L426 L427 L428 L429 L430
